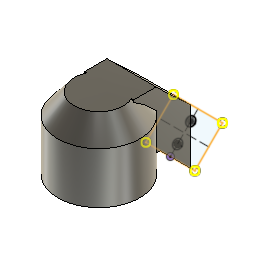
RT24_CapsChannel (Autodesk Fusion 360 design; units mm, degrees)
Autodesk Fusion 360 part; units mm, degrees
note: some values were not read from the file. Chosen so that the rebuilt part matches the saved one: which face or edge a step refers to.
sketch "Sketch1" plane through (0, 0, 0) normal (1, 0, 0) x (0, 1, 0)
  line L0 (0, 20) -> (5, 20)
  line L1 (5, 20) -> (5, 17)
  line L2 (5, 17) -> (7.5, 17)
  line L3 (7.5, 17) -> (7.5, 8)
  line L4 (0, 23) -> (6, 23)
  line L5 (6, 23) -> (10, 18)
  line L6 (10, 18) -> (10, 8)
  line L7 (10, 8) -> (7.5, 8)
  line L8 (0, 20) -> (0, 23)
  line L9 (0, 20) -> (0, 8)
  line L10 (0, 8) -> (7.5, 8)
  line L11 (10, 8) -> (10, 5.5)
  line L12 (10, 5.5) -> (0, 5.5)
  line L13 (0, 5.5) -> (0, 8)
  line L14 (7.5, 8) -> (7.8879, 5.5)
  dimension "d1" = 5
  dimension "d2" = 20
  dimension "d57" = 2.5
  constraint horizontal L0
  constraint perpendicular L0 L1
  constraint perpendicular L1 L2
  constraint perpendicular L2 L3
  constraint parallel L0 L4
  constraint perpendicular L4 L6
  constraint perpendicular L4 L8
  constraint perpendicular L0 L9
  constraint perpendicular L7 L11
  constraint perpendicular L9 L12
  constraint parallel L9 L13
  constraint coincident L12 L14.end
  measures "d1" distance of L0.start L0.end
  measures "d2" distance of origin L0.start
  measures "d57" distance of L6.end L11.end
revolve "Revolve1" add sketch "Sketch1" angle 360 about axis through (0, 0, 1.75) along (0, 0, 1) contours L0 L1 L2 L3 L4 L5 L6 L7 L8 | L7 L11 L12 L14
sketch "Sketch2" plane through (0, 0, 8) normal (0, 0, -1) x (1, 0, 0)
  circle A0 centre (0, 0) radius 10
  circle A1 centre (0, 0) radius 7.5
  line L0 (0, 0) -> (-15, 0) construction
  line L1 (0, 0) -> (15, 0) construction
  circle A2 centre (-15, 0) radius 6.75
  circle A3 centre (15, 0) radius 6.75
  line L2 (-15.0149, -6.75) -> (-15.0149, 6.75)
  line L3 (15, -8.5) -> (15, 8.5)
  dimension "d16" = 13.5
  dimension "d17" = 13.5
  dimension "d41" = 15
  constraint coincident A0.centre A1.centre
  constraint horizontal L0
  constraint parallel L0 L1
  constraint coincident L0.end A2.centre
  constraint coincident L1.end A3.centre
  constraint coincident A2 L2.start
  constraint coincident A2 L2.end
  constraint perpendicular L0 L2
  constraint vertical L3
  measures "d16" diameter of A2
  measures "d17" diameter of A3
  measures "d41" distance of A0.centre L1.end
sketch "Sketch3" plane through (0, 0, 0) normal (0, 1, 0) x (1, 0, 0)
  line L0 (-15, -8) -> (-15, -15.1623)
  spline S0 degree 5 poles (-15, -15.1623) (-15, -15.5572) (-15.0542, -16.279) (-15.2979, -17.1585) (-15.8999, -17.9784) (-16.9384, -18.5963) (-17.8782, -18.8676) (-18.6005, -18.9696) (-19.0851, -18.9923) (-19.3282, -18.9923) knots 0 0 0 0 0 0 0.2 0.4 0.6 0.8 1 1 1 1 1 1
  line L1 (-18.689, -18.9923) -> (-19.9674, -18.9923)
  line L2 (-15, -14.1623) -> (-15, -16.1623)
  line L3 (0, -35) -> (0, 0) construction
  spline S1 degree 5 poles (15, -15.1623) (15, -15.5572) (15.0542, -16.279) (15.2979, -17.1585) (15.8999, -17.9784) (16.9384, -18.5963) (17.8782, -18.8676) (18.6005, -18.9696) (19.0851, -18.9923) (19.3282, -18.9923) knots 0 0 0 0 0 0 0.2 0.4 0.6 0.8 1 1 1 1 1 1
  line L4 (15, -14.1623) -> (15, -16.1623)
  line L5 (18.689, -18.9923) -> (19.9674, -18.9923)
  line L6 (15, -8) -> (15, -15.1623)
  line L7 (-15, -8) -> (-15, 0)
  line L8 (15, -8) -> (15, 0)
  point P0 (15, -8)
  point P1 (-15, -8)
  constraint coincident P1 L0.start
  constraint vertical L0
  constraint midpoint S0.end L1
  constraint midpoint L0.end L2
  constraint coincident L0 L2.start
  constraint coincident L3.end origin
  constraint vertical L3
  constraint symmetric P1 L3 P0
  constraint symmetric L0.end L3 S1.start
  constraint symmetric S0.end L3 S1.end
  constraint symmetric L1.start L3 L5.start
  constraint symmetric L1.end L3 L5.end
  constraint symmetric L2.start L3 L4.start
  constraint symmetric L2.end L3 L4.end
  constraint parallel L0 L7
  constraint coincident P0 L6.start
  constraint parallel L6 L8
sweep "Sweep1" cut profiles "Sketch2" path "Sketch3" along L7 L0 S0 section 1 contours A0 A2 | A0 A2 L2
sketch "Sketch4" plane through (0, 0, 0) normal (1, 0, 0) x (0, 1, 0)
  line L0 (9, 9) -> (17.4853, 0.5147)
  line L1 (17.4853, 0.5147) -> (17.4853, 14)
  line L2 (5, 9) -> (9, 9)
  line L3 (5, 9) -> (2.5, 23)
  line L4 (9, 22) -> (17.4853, 14)
  line L5 (2.5, 23) -> (8, 23)
  line L6 (8, 23) -> (9, 22)
  line L7 (16.5, 1.5) -> (16.5, 15.784)
  dimension "d23" = 12
  constraint vertical L1
  constraint horizontal L5
  constraint coincident L0 L7.start
  constraint parallel L1 L7
  measures "d23" distance of L0.start L0.end
extrude "Extrude1" add sketch "Sketch4" along normal mid plane 12 contours L0 L2 L3 L4 L5 L6 L7
ref_plane "WorkPlane1" through (0, 17.4853, 0.5147) normal (0, -0.707107, 0.707107) x (1, 0, 0)
sketch "Sketch5" plane through (0, 17.4853, 0.5147) normal (0, -0.707107, 0.707107) x (1, 0, 0)
  line L0 (-6, 0) -> (-6, 9.5355)
  line L1 (-6, 9.5355) -> (6, 9.5355)
  line L2 (6, 9.5355) -> (6, 0)
  line L3 (6, 0) -> (-6, 0)
  line L4 (6, 4.7678) -> (-6, 4.7678) construction
  line L5 (0, 0) -> (0, 9.5355) construction
  circle A0 centre (0, 2.5) radius 1
  circle A1 centre (0, 7.0355) radius 1
  dimension "d35" = 9.5355
  dimension "d36" = 2
  dimension "d37" = 2.5
  constraint midpoint L2 L4.start
  constraint midpoint L0 L4.end
  constraint coincident L5.start origin
  constraint midpoint L1 L5.end
  constraint coincident L5 A0.centre
  constraint symmetric L4 A0 A1
  measures "d35" distance of L5.start L5.end
  measures "d36" diameter of A0
  measures "d37" distance of L3 A0.centre
revolve "Revolve2" [suppressed]
ref_plane "WorkPlane2" through (0, 0, 12.125) normal (-0.052336, 0.99863, 0) x (0, 0, 1)
sketch "Sketch6" plane through (0, 0, 12.125) normal (-0.052336, 0.99863, 0) x (0, 0, 1)
  line L0 (-4.125, 14.9794) -> (3.0373, 14.9794)
  spline S0 degree 5 poles (3.0373, 14.9794) (3.4322, 14.9794) (4.154, 15.0336) (5.0335, 15.277) (5.8534, 15.8782) (6.4713, 16.9152) (6.7426, 17.8537) (6.8446, 18.575) (6.8673, 19.059) (6.8673, 19.3017) knots 0 0 0 0 0 0 0.2 0.4 0.6 0.8 1 1 1 1 1 1
  line L1 (-4.125, 14.9794) -> (-12.125, 14.9794)
ref_plane "WorkPlane3" through (0, 0, 8) normal (0, 0, -1) x (-1, 0, 0)
sketch "Sketch7" plane through (0, 5.5565, 8) normal (0, 0, -1) x (1, 0, 0)
  circle A0 centre (14.9589, 4.7725) radius 6.75
  line L0 (16.1557, 11.4156) -> (14.9589, 4.7725)
  line L1 (14.9589, 4.7725) -> (13.7621, -1.8705)
  point P0 (14.9589, 4.7725)
  dimension "d44" = 13.5
  constraint coincident P0 A0.centre
  constraint coincident A0 L0.start
  constraint coincident A0 L1.end
  constraint parallel L0 L1
  measures "d44" diameter of A0
sweep "Sweep3" [suppressed]
ref_plane "WorkPlane4" through (0, 17.4853, 0.5147) normal (0, 0, 1) x (1, 0, 0)
sketch "Sketch8" plane through (0, 17.4853, 0.5147) normal (0, 0, 1) x (1, 0, 0)
  arc A0 (4.3589, -8.4853) -> (-4.3589, -8.4853) centre (0, -17.4853) ccw
  line L0 (-4.3589, -8.4853) -> (-6, -8.4853)
  line L1 (-6, -8.4853) -> (-6, -0.9853)
  line L2 (6, -0.9853) -> (6, -8.4853)
  line L3 (-6, -3) -> (6, -3)
  line L4 (6, -8.4853) -> (4.3589, -8.4853)
  line L5 (-6, -0.9853) -> (6, -0.9853)
  constraint coincident L1 L3.start
  constraint coincident L2 L3.end
  constraint perpendicular L2 L3
extrude "Extrude3" [suppressed]
fillet "Fillet4" [suppressed]
extrude "Extrude4" [suppressed]
